Autodesk Inventor part; units mm, degrees
(part 2 of 2)
sketch "Sketch5" plane through (0, 1.5, 0) normal (0, 1, 0) x (1, 0, 0)
  line L0 (-89.6198, -3.6421) -> (-89.6198, 518.675) construction
  line L1 (-89.6198, 518.675) -> (-0.3513, 518.675) construction
  line L2 (-0.3513, 518.675) -> (-0.3513, -3.6421) construction
  line L3 (-0.3513, -3.6421) -> (-89.6198, -3.6421) construction
  spline S0 degree 2 poles (-71.9836, 45.1863) (-68.0845, 45.1863) (-61.0119, 42.6927) (-58.6544, 40.3805) knots 0 0 0 1 2 2 2
  spline S1 degree 2 poles (-58.6544, 40.3805) (-57.1582, 38.9751) (-54.71, 35.5294) (-53.8486, 33.4893) knots 0 0 0 1 2 2 2
  spline S2 degree 2 poles (-53.8486, 33.4893) (-52.9872, 31.4037) (-51.9898, 26.5526) (-51.9898, 23.5604) knots 0 0 0 1 2 2 2
  line L4 (-51.9898, 23.5604) -> (-51.9898, 16.2157)
  line L5 (-51.9898, 16.2157) -> (-33.6735, 16.2157)
  line L6 (-33.6735, 16.2157) -> (-33.6735, 2.1611)
  line L7 (-33.6735, 2.1611) -> (-89.6198, 2.1611)
  line L8 (-89.6198, 2.1611) -> (-89.6198, 23.8777)
  spline S3 degree 2 poles (-89.6198, 23.8777) (-89.6198, 28.6835) (-87.8516, 35.7108) (-85.9475, 38.567) knots 0 0 0 1 2 2 2
  spline S4 degree 2 poles (-85.9475, 38.567) (-83.8166, 41.7407) (-76.8347, 45.1863) (-71.9836, 45.1863) knots 0 0 0 1 2 2 2
  spline S5 degree 2 poles (-71.6209, 30.769) (-74.0237, 30.769) (-77.424, 28.5021) (-78.0588, 26.9607) knots 0 0 0 1 2 2 2
  spline S6 degree 2 poles (-78.0588, 26.9607) (-78.9202, 24.9658) (-79.1922, 21.3388) (-79.1922, 18.2106) knots 0 0 0 1 2 2 2
  line L9 (-79.1922, 18.2106) -> (-79.1922, 16.2157)
  line L10 (-79.1922, 16.2157) -> (-62.4174, 16.2157)
  line L11 (-62.4174, 16.2157) -> (-62.4174, 17.2131)
  spline S7 degree 2 poles (-62.4174, 17.2131) (-62.4174, 19.1626) (-62.508, 22.699) (-62.7347, 24.0137) knots 0 0 0 1 2 2 2
  spline S8 degree 2 poles (-62.7347, 24.0137) (-62.9161, 25.1472) (-64.0042, 27.6407) (-64.6842, 28.3208) knots 0 0 0 1 2 2 2
  spline S9 degree 2 poles (-64.6842, 28.3208) (-66.0444, 29.7716) (-69.082, 30.769) (-71.6209, 30.769) knots 0 0 0 1 2 2 2
  line L12 (-33.6735, 126.9296) -> (-33.6735, 109.8374)
  line L13 (-33.6735, 109.8374) -> (-54.2113, 94.2867)
  line L14 (-54.2113, 94.2867) -> (-54.2113, 89.2089)
  line L15 (-54.2113, 89.2089) -> (-33.6735, 89.2089)
  line L16 (-33.6735, 89.2089) -> (-33.6735, 75.245)
  line L17 (-33.6735, 75.245) -> (-89.6198, 75.245)
  line L18 (-89.6198, 75.245) -> (-89.6198, 97.7323)
  spline S10 degree 2 poles (-89.6198, 97.7323) (-89.6198, 102.4021) (-88.441, 109.2934) (-86.6275, 112.2403) knots 0 0 0 1 2 2 2
  spline S11 degree 2 poles (-86.6275, 112.2403) (-84.7234, 115.2325) (-78.7842, 118.7689) (-74.2504, 118.7689) knots 0 0 0 1 2 2 2
  spline S12 degree 2 poles (-74.2504, 118.7689) (-67.8579, 118.7689) (-59.8331, 112.9657) (-57.4756, 108.1146) knots 0 0 0 1 2 2 2
  line L19 (-57.4756, 108.1146) -> (-33.6735, 126.9296)
  spline S13 degree 2 poles (-72.4823, 104.3516) (-74.6131, 104.3516) (-77.6507, 102.7194) (-78.4668, 100.8606) knots 0 0 0 1 2 2 2
  spline S14 degree 2 poles (-78.4668, 100.8606) (-79.0108, 99.5458) (-79.3282, 96.3269) (-79.3282, 93.924) knots 0 0 0 1 2 2 2
  line L20 (-79.3282, 93.924) -> (-79.3282, 89.2089)
  line L21 (-79.3282, 89.2089) -> (-64.2762, 89.2089)
  line L22 (-64.2762, 89.2089) -> (-64.2762, 93.2439)
  spline S15 degree 2 poles (-64.2762, 93.2439) (-64.2762, 96.1455) (-65.0016, 100.2712) (-66.135, 101.6767) knots 0 0 0 1 2 2 2
  spline S16 degree 2 poles (-66.135, 101.6767) (-67.2231, 103.0368) (-70.1247, 104.3516) (-72.4823, 104.3516) knots 0 0 0 1 2 2 2
  line L23 (-33.6735, 181.4705) -> (-33.6735, 151.3664)
  line L24 (-33.6735, 151.3664) -> (-43.421, 151.3664)
  line L25 (-43.421, 151.3664) -> (-43.421, 159.3912)
  line L26 (-43.421, 159.3912) -> (-79.8723, 159.3912)
  line L27 (-79.8723, 159.3912) -> (-79.8723, 151.3664)
  line L28 (-79.8723, 151.3664) -> (-89.6198, 151.3664)
  line L29 (-89.6198, 151.3664) -> (-89.6198, 181.4705)
  line L30 (-89.6198, 181.4705) -> (-79.8723, 181.4705)
  line L31 (-79.8723, 181.4705) -> (-79.8723, 173.4457)
  line L32 (-79.8723, 173.4457) -> (-43.421, 173.4457)
  line L33 (-43.421, 173.4457) -> (-43.421, 181.4705)
  line L34 (-43.421, 181.4705) -> (-33.6735, 181.4705)
  spline S17 degree 2 poles (-61.6013, 263.2591) (-53.7579, 263.2591) (-41.4262, 256.4131) (-38.1165, 251.1994) knots 0 0 0 1 2 2 2
  spline S18 degree 2 poles (-38.1165, 251.1994) (-35.3056, 246.847) (-33.6735, 236.6007) (-33.6735, 230.8429) knots 0 0 0 1 2 2 2
  line L35 (-33.6735, 230.8429) -> (-33.6735, 213.3426)
  line L36 (-33.6735, 213.3426) -> (-89.6198, 213.3426)
  line L37 (-89.6198, 213.3426) -> (-89.6198, 230.6615)
  spline S19 degree 2 poles (-89.6198, 230.6615) (-89.6198, 236.5554) (-88.1237, 246.847) (-85.2221, 251.3807) knots 0 0 0 1 2 2 2
  spline S20 degree 2 poles (-85.2221, 251.3807) (-81.6858, 256.8665) (-69.7167, 263.2591) (-61.6013, 263.2591) knots 0 0 0 1 2 2 2
  spline S21 degree 2 poles (-61.692, 248.8418) (-67.2231, 248.8418) (-75.1118, 245.0335) (-77.3334, 241.1345) knots 0 0 0 1 2 2 2
  spline S22 degree 2 poles (-77.3334, 241.1345) (-78.8748, 238.2782) (-79.1922, 232.0216) (-79.1922, 227.6693) knots 0 0 0 1 2 2 2
  line L38 (-79.1922, 227.6693) -> (-79.1922, 227.3972)
  line L39 (-79.1922, 227.3972) -> (-44.1464, 227.3972)
  line L40 (-44.1464, 227.3972) -> (-44.1464, 227.6693)
  spline S23 degree 2 poles (-44.1464, 227.6693) (-44.1464, 232.3843) (-44.4638, 238.8676) (-46.3226, 241.8145) knots 0 0 0 1 2 2 2
  spline S24 degree 2 poles (-46.3226, 241.8145) (-48.4988, 245.2602) (-56.1608, 248.8418) (-61.692, 248.8418) knots 0 0 0 1 2 2 2
  line L41 (-33.6735, 294.1338) -> (-89.6198, 294.1338)
  line L42 (-89.6198, 294.1338) -> (-89.6198, 331.9452)
  line L43 (-89.6198, 331.9452) -> (-78.9655, 331.9452)
  line L44 (-78.9655, 331.9452) -> (-78.9655, 308.0978)
  line L45 (-78.9655, 308.0978) -> (-69.1273, 308.0978)
  line L46 (-69.1273, 308.0978) -> (-69.1273, 330.0864)
  line L47 (-69.1273, 330.0864) -> (-58.473, 330.0864)
  line L48 (-58.473, 330.0864) -> (-58.473, 308.0978)
  line L49 (-58.473, 308.0978) -> (-44.3278, 308.0978)
  line L50 (-44.3278, 308.0978) -> (-44.3278, 331.9452)
  line L51 (-44.3278, 331.9452) -> (-33.6735, 331.9452)
  line L52 (-33.6735, 331.9452) -> (-33.6735, 294.1338)
  point P0 (0, 0)
  constraints: 2 other
extrude "Extrusion5" cut sketch "Sketch5" against normal blind 0.2
body "Solid1"
